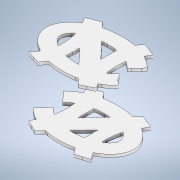
# Autodesk Inventor part: HousingLogoPositive
Saved by Autodesk Inventor 2020 (Build 240168000, 168)
## iProperties
Created: 2019-09-04
Part Number: HousingLogoPositive
Material: Generic
Document SubType Name: Modeling
Designer: Eric
Density: 1 g/cm^3
Appearance: White
Author: Eric
Autodesk Inventor part; units mm, degrees
note: some values were not read from the file. Chosen so that the rebuilt part matches the saved one: direction of "Hole1"; direction of "Hole2".
(part 1 of 2)
sketch "Sketch1" plane through (0, 0, 0) normal (0, 0, 1) x (1, 0, 0)
  arc A0 (31.8897, -7.6835) -> (33.4645, -6.1087) centre (31.8897, -6.1087) ccw projected
  line L0 (33.4645, 6.1087) -> (33.4645, -6.1087) projected
  arc A1 (33.4645, 6.1087) -> (31.8897, 7.6835) centre (31.8897, 6.1087) ccw projected
  line L1 (-31.8897, 7.6835) -> (31.8897, 7.6835) projected
  arc A2 (-31.8897, 7.6835) -> (-33.4645, 6.1087) centre (-31.8897, 6.1087) ccw projected
  line L2 (-33.4645, -6.1087) -> (-33.4645, 6.1087) projected
  arc A3 (-33.4645, -6.1087) -> (-31.8897, -7.6835) centre (-31.8897, -6.1087) ccw projected
  line L3 (31.8897, -7.6835) -> (-31.8897, -7.6835) projected
  circle A4 centre (-30.5562, 0) radius 1.524 projected
  circle A5 centre (30.5562, 0) radius 1.524 projected
  arc A6 (-24.5555, 6.9912) -> (-27.8573, 3.0561) centre (-24.5555, 3.6383) ccw projected
  line L4 (24.5555, 6.9912) -> (-24.5555, 6.9912) projected
  arc A7 (27.8573, 3.0561) -> (24.5555, 6.9912) centre (24.5555, 3.6383) ccw projected
  line L5 (26.5742, -4.2206) -> (27.8573, 3.0561) projected
  arc A8 (23.2724, -6.9912) -> (26.5742, -4.2206) centre (23.2724, -3.6383) ccw projected
  line L6 (-23.2724, -6.9912) -> (23.2724, -6.9912) projected
  arc A9 (-26.5742, -4.2206) -> (-23.2724, -6.9912) centre (-23.2724, -3.6383) ccw projected
  line L7 (-27.8573, 3.0561) -> (-26.5742, -4.2206) projected
  arc A10 (37.0645, 6.1087) -> (31.8897, 11.2835) centre (31.8897, 6.1087) ccw
  line L8 (37.0645, 6.1087) -> (37.0645, -6.1087)
  arc A11 (31.8897, -11.2835) -> (37.0645, -6.1087) centre (31.8897, -6.1087) ccw
  line L9 (31.8897, -11.2835) -> (-31.8897, -11.2835)
  arc A12 (-37.0645, -6.1087) -> (-31.8897, -11.2835) centre (-31.8897, -6.1087) ccw
  line L10 (-37.0645, -6.1087) -> (-37.0645, 6.1087)
  arc A13 (-31.8897, 11.2835) -> (-37.0645, 6.1087) centre (-31.8897, 6.1087) ccw
  line L11 (-31.8897, 11.2835) -> (31.8897, 11.2835)
  arc A14 (-24.5555, 7.3911) -> (-28.2512, 2.9867) centre (-24.5555, 3.6383) ccw
  line L12 (-24.5555, 7.3911) -> (24.5555, 7.3912)
  arc A15 (28.2512, 2.9867) -> (24.5555, 7.3912) centre (24.5555, 3.6383) ccw
  line L13 (28.2512, 2.9867) -> (26.9682, -4.29)
  arc A16 (23.2724, -7.3911) -> (26.9682, -4.29) centre (23.2724, -3.6383) ccw
  line L14 (23.2724, -7.3911) -> (-23.2724, -7.3912)
  arc A17 (-26.9682, -4.29) -> (-23.2724, -7.3912) centre (-23.2724, -3.6383) ccw
  line L15 (-26.9682, -4.29) -> (-28.2512, 2.9867)
  point P0 (0, 0)
  dimension "d0" = 3.6
  dimension "d1" = 0.4
  constraints: 16 end point, 16 point on circle, 8 centre point, 14 other
  measures "d0" distance between parallel lines of L1 L11
  measures "d1" distance between parallel lines of L4 L12
extrude "Extrusion1" add sketch "Sketch1" along normal blind 1.2 contours L3 A3 L2 A2 L1 A1 L0 A0 | L8 A11 L9 A12 L10 A13 L11 A10
sketch "Sketch2" plane through (0, 0, 0) normal (0, 0, -1) x (-1, 0, 0)
  arc A0 (-33.4645, -6.1087) -> (-31.8897, -7.6835) centre (-31.8897, -6.1087) ccw projected
  line L0 (-33.4645, 6.1087) -> (-33.4645, -6.1087) projected
  arc A1 (-31.8897, 7.6835) -> (-33.4645, 6.1087) centre (-31.8897, 6.1087) ccw projected
  line L1 (31.8897, 7.6835) -> (-31.8897, 7.6835) projected
  arc A2 (33.4645, 6.1087) -> (31.8897, 7.6835) centre (31.8897, 6.1087) ccw projected
  line L2 (33.4645, -6.1087) -> (33.4645, 6.1087) projected
  arc A3 (31.8897, -7.6835) -> (33.4645, -6.1087) centre (31.8897, -6.1087) ccw projected
  line L3 (-31.8897, -7.6835) -> (31.8897, -7.6835) projected
  circle A4 centre (30.5562, 0) radius 1.524 projected
  circle A5 centre (-30.5562, 0) radius 1.524 projected
  arc A6 (27.8573, 3.0561) -> (24.5555, 6.9912) centre (24.5555, 3.6383) ccw projected
  line L4 (-24.5555, 6.9912) -> (24.5555, 6.9912) projected
  arc A7 (-24.5555, 6.9912) -> (-27.8573, 3.0561) centre (-24.5555, 3.6383) ccw projected
  line L5 (-26.5742, -4.2206) -> (-27.8573, 3.0561) projected
  arc A8 (-26.5742, -4.2206) -> (-23.2724, -6.9912) centre (-23.2724, -3.6383) ccw projected
  line L6 (23.2724, -6.9912) -> (-23.2724, -6.9912) projected
  arc A9 (23.2724, -6.9912) -> (26.5742, -4.2206) centre (23.2724, -3.6383) ccw projected
  line L7 (27.8573, 3.0561) -> (26.5742, -4.2206) projected
  line L8 (37.0645, 6.1087) -> (37.0645, -6.1087) projected
  arc A10 (37.0645, 6.1087) -> (31.8897, 11.2835) centre (31.8897, 6.1087) ccw projected
  line L9 (-31.8897, 11.2835) -> (31.8897, 11.2835) projected
  arc A11 (-31.8897, 11.2835) -> (-37.0645, 6.1087) centre (-31.8897, 6.1087) ccw projected
  line L10 (-37.0645, -6.1087) -> (-37.0645, 6.1087) projected
  arc A12 (-37.0645, -6.1087) -> (-31.8897, -11.2835) centre (-31.8897, -6.1087) ccw projected
  line L11 (31.8897, -11.2835) -> (-31.8897, -11.2835) projected
  arc A13 (31.8897, -11.2835) -> (37.0645, -6.1087) centre (31.8897, -6.1087) ccw projected
  arc A14 (28.2512, 2.9867) -> (24.5555, 7.3911) centre (24.5555, 3.6383) ccw projected
  line L12 (26.9682, -4.29) -> (28.2512, 2.9867) projected
  arc A15 (23.2724, -7.3912) -> (26.9682, -4.29) centre (23.2724, -3.6383) ccw projected
  line L13 (-23.2724, -7.3911) -> (23.2724, -7.3912) projected
  arc A16 (-26.9682, -4.29) -> (-23.2724, -7.3911) centre (-23.2724, -3.6383) ccw projected
  line L14 (-28.2512, 2.9867) -> (-26.9682, -4.29) projected
  arc A17 (-24.5555, 7.3912) -> (-28.2512, 2.9867) centre (-24.5555, 3.6383) ccw projected
  line L15 (24.5555, 7.3911) -> (-24.5555, 7.3912) projected
  circle A18 centre (-30.5562, 0) radius 1.524 projected
  circle A19 centre (30.5562, 0) radius 1.524 projected
  arc A20 (-31.8897, 8.0835) -> (-33.8645, 6.1087) centre (-31.8897, 6.1087) ccw
  line L16 (-33.8645, 6.1087) -> (-33.8645, -6.1087)
  arc A21 (-33.8645, -6.1087) -> (-31.8897, -8.0835) centre (-31.8897, -6.1087) ccw
  line L17 (-31.8897, -8.0835) -> (31.8897, -8.0835)
  arc A22 (31.8897, -8.0835) -> (33.8645, -6.1087) centre (31.8897, -6.1087) ccw
  line L18 (33.8645, -6.1087) -> (33.8645, 6.1087)
  arc A23 (33.8645, 6.1087) -> (31.8897, 8.0835) centre (31.8897, 6.1087) ccw
  line L19 (31.8897, 8.0835) -> (-31.8897, 8.0835)
  point P0 (0, 0)
  dimension "d4" = 0.4
  constraints: 8 end point, 8 point on circle, 4 centre point, 7 other
  measures "d4" distance between parallel lines of L1 L19
extrude "Extrusion2" add sketch "Sketch2" along normal blind 1.6 contours L8 A13 L11 A12 L10 A11 L9 A10
sketch "Sketch3" plane through (0, 0, -1.6) normal (0, 0, -1) x (-1, 0, 0)
  line L0 (31.8897, 11.2835) -> (-31.8897, 11.2835) projected
  arc A0 (-31.8897, 11.2835) -> (-37.0645, 6.1087) centre (-31.8897, 6.1087) ccw projected
  line L1 (-37.0645, 6.1087) -> (-37.0645, -6.1087) projected
  arc A1 (-37.0645, -6.1087) -> (-31.8897, -11.2835) centre (-31.8897, -6.1087) ccw projected
  line L2 (-31.8897, -11.2835) -> (31.8897, -11.2835) projected
  arc A2 (31.8897, -11.2835) -> (37.0645, -6.1087) centre (31.8897, -6.1087) ccw projected
  line L3 (37.0645, -6.1087) -> (37.0645, 6.1087) projected
  arc A3 (37.0645, 6.1087) -> (31.8897, 11.2835) centre (31.8897, 6.1087) ccw projected
  arc A4 (-31.8897, 8.0835) -> (-33.8645, 6.1087) centre (-31.8897, 6.1087) ccw projected
  line L4 (-31.8897, 8.0835) -> (31.8897, 8.0835) projected
  arc A5 (33.8645, 6.1087) -> (31.8897, 8.0835) centre (31.8897, 6.1087) ccw projected
  line L5 (33.8645, 6.1087) -> (33.8645, -6.1087) projected
  arc A6 (31.8897, -8.0835) -> (33.8645, -6.1087) centre (31.8897, -6.1087) ccw projected
  line L6 (31.8897, -8.0835) -> (-31.8897, -8.0835) projected
  arc A7 (-33.8645, -6.1087) -> (-31.8897, -8.0835) centre (-31.8897, -6.1087) ccw projected
  line L7 (-33.8645, -6.1087) -> (-33.8645, 6.1087) projected
  circle A8 centre (-30.5562, 0) radius 1.524 projected
  line L8 (37.0645, 6.1087) -> (37.0645, -6.1087) projected
  arc A9 (31.8897, -11.2835) -> (37.0645, -6.1087) centre (31.8897, -6.1087) ccw projected
  line L9 (31.8897, -11.2835) -> (-31.8897, -11.2835) projected
  arc A10 (-37.0645, -6.1087) -> (-31.8897, -11.2835) centre (-31.8897, -6.1087) ccw projected
  line L10 (-37.0645, -6.1087) -> (-37.0645, 6.1087) projected
  arc A11 (-31.8897, 11.2835) -> (-37.0645, 6.1087) centre (-31.8897, 6.1087) ccw projected
  line L11 (-31.8897, 11.2835) -> (31.8897, 11.2835) projected
  arc A12 (37.0645, 6.1087) -> (31.8897, 11.2835) centre (31.8897, 6.1087) ccw projected
  arc A13 (28.2512, 2.9867) -> (24.5555, 7.3911) centre (24.5555, 3.6383) ccw projected
  line L12 (24.5555, 7.3911) -> (-24.5555, 7.3912) projected
  arc A14 (-24.5555, 7.3912) -> (-28.2512, 2.9867) centre (-24.5555, 3.6383) ccw projected
  line L13 (-28.2512, 2.9867) -> (-26.9682, -4.29) projected
  arc A15 (-26.9682, -4.29) -> (-23.2724, -7.3911) centre (-23.2724, -3.6383) ccw projected
  line L14 (-23.2724, -7.3911) -> (23.2724, -7.3912) projected
  arc A16 (23.2724, -7.3912) -> (26.9682, -4.29) centre (23.2724, -3.6383) ccw projected
  line L15 (26.9682, -4.29) -> (28.2512, 2.9867) projected
  circle A17 centre (-30.5562, 0) radius 1.524 projected
  circle A18 centre (30.5562, 0) radius 1.524 projected
  line L16 (-31.8897, -8.0835) -> (31.8897, -8.0835) projected
  arc A19 (28.2512, 2.9867) -> (24.5555, 7.3911) centre (24.5555, 3.6383) ccw projected
  line L17 (-23.2724, -7.3911) -> (23.2724, -7.3912) projected
  arc A20 (23.2724, -7.3912) -> (26.9682, -4.29) centre (23.2724, -3.6383) ccw projected
  point P0 (0, 0)
ref_plane "Work Plane1" through (20.4432, -5.693, -21.5638) normal (0, 0, 1) x (1, 0, 0)
extrude "Extrusion3" add sketch "Sketch3" along normal up to surface (19.9638 mm away) contours A3 L3 A2 L2 A1 L1 A0 L0 | L4 A5 L5 A6 L6 A7 L7 A4
sketch "Sketch4" plane through (31.8897, -11.2835, -21.5638) normal (0, 0, -1) x (-1, 0, 0)
  circle A0 centre (1.3335, 11.2835) radius 1.524 projected
  circle A1 centre (62.4459, 11.2835) radius 1.524 projected
  point P0 (31.8897, 11.2835)
  constraints: 2 coincident
hole "Hole1" at (-30.5562, 0, -21.5638) at (30.5562, 0, -21.5638) direction (0, 0, 1) diameter 3.2 depth 19.9638
ref_plane "Work Plane2" through (-21.3801, -2.5043, -26.2897) normal (0, -0.0871557, -0.9961947) x (1, 0, 0)
sketch "Sketch6" plane through (-21.3801, -2.5043, -26.2897) normal (0, -0.0871557, -0.9961947) x (1, 0, 0)
  arc A0 (-0.0392, 3.5884) -> (-0.8476, 1.4884) centre (1.375, 1.8384) ccw projected
  line L0 (-0.8476, 1.4884) -> (-0.325, 1.4884) projected
  line L1 (-0.325, 1.4884) -> (-0.325, 0.4134) projected
  line L2 (-0.325, 0.4134) -> (0, 0.0884) projected
  line L3 (0, 0.0884) -> (2.75, 0.0884) projected
  line L4 (2.75, 0.0884) -> (3.075, 0.4134) projected
  line L5 (3.075, 0.4134) -> (3.075, 1.4884) projected
  line L6 (3.075, 1.4884) -> (3.5976, 1.4884) projected
  arc A1 (3.5976, 1.4884) -> (2.7892, 3.5884) centre (1.375, 1.8384) ccw projected
  line L7 (-0.0392, 3.5884) -> (2.7892, 3.5884) projected
  circle A2 centre (1.375, 1.8384) radius 1.55 projected
  arc A3 (7.6685, -1.9054) -> (8.4769, 0.1946) centre (6.2543, -0.1554) ccw projected
  line L8 (8.4769, 0.1946) -> (7.9543, 0.1946) projected
  line L9 (7.9543, 0.1946) -> (7.9543, 1.2696) projected
  line L10 (7.9543, 1.2696) -> (7.6293, 1.5946) projected
  line L11 (7.6293, 1.5946) -> (4.8793, 1.5946) projected
  line L12 (4.8793, 1.5946) -> (4.5543, 1.2696) projected
  line L13 (4.5543, 1.2696) -> (4.5543, 0.1946) projected
  line L14 (4.5543, 0.1946) -> (4.0316, 0.1946) projected
  arc A4 (4.0316, 0.1946) -> (4.84, -1.9054) centre (6.2543, -0.1554) ccw projected
  line L15 (7.6685, -1.9054) -> (4.84, -1.9054) projected
  circle A5 centre (6.2543, -0.1554) radius 1.55 projected
  arc A6 (9.7193, 3.5884) -> (8.9109, 1.4884) centre (11.1335, 1.8384) ccw projected
  line L16 (8.9109, 1.4884) -> (9.4335, 1.4884) projected
  line L17 (9.4335, 1.4884) -> (9.4335, 0.4134) projected
  line L18 (9.4335, 0.4134) -> (9.7585, 0.0884) projected
  line L19 (9.7585, 0.0884) -> (12.5085, 0.0884) projected
  line L20 (12.5085, 0.0884) -> (12.8335, 0.4134) projected
  line L21 (12.8335, 0.4134) -> (12.8335, 1.4884) projected
  line L22 (12.8335, 1.4884) -> (13.3561, 1.4884) projected
  arc A7 (13.3561, 1.4884) -> (12.5477, 3.5884) centre (11.1335, 1.8384) ccw projected
  line L23 (9.7193, 3.5884) -> (12.5477, 3.5884) projected
  circle A8 centre (11.1335, 1.8384) radius 1.55 projected
  arc A9 (17.427, -1.9054) -> (18.2354, 0.1946) centre (16.0128, -0.1554) ccw projected
  line L24 (18.2354, 0.1946) -> (17.7128, 0.1946) projected
  line L25 (17.7128, 0.1946) -> (17.7128, 1.2696) projected
  line L26 (17.7128, 1.2696) -> (17.3878, 1.5946) projected
  line L27 (17.3878, 1.5946) -> (14.6378, 1.5946) projected
  line L28 (14.6378, 1.5946) -> (14.3128, 1.2696) projected
  line L29 (14.3128, 1.2696) -> (14.3128, 0.1946) projected
  line L30 (14.3128, 0.1946) -> (13.7902, 0.1946) projected
  arc A10 (13.7902, 0.1946) -> (14.5986, -1.9054) centre (16.0128, -0.1554) ccw projected
  line L31 (17.427, -1.9054) -> (14.5986, -1.9054) projected
  circle A11 centre (16.0128, -0.1554) radius 1.55 projected
  arc A12 (19.4778, 3.5884) -> (18.6694, 1.4884) centre (20.892, 1.8384) ccw projected
  line L32 (18.6694, 1.4884) -> (19.192, 1.4884) projected
  line L33 (19.192, 1.4884) -> (19.192, 0.4134) projected
  line L34 (19.192, 0.4134) -> (19.517, 0.0884) projected
  line L35 (19.517, 0.0884) -> (22.267, 0.0884) projected
  line L36 (22.267, 0.0884) -> (22.592, 0.4134) projected
  line L37 (22.592, 0.4134) -> (22.592, 1.4884) projected
  line L38 (22.592, 1.4884) -> (23.1147, 1.4884) projected
  arc A13 (23.1147, 1.4884) -> (22.3063, 3.5884) centre (20.892, 1.8384) ccw projected
  line L39 (19.4778, 3.5884) -> (22.3063, 3.5884) projected
  circle A14 centre (20.892, 1.8384) radius 1.55 projected
  arc A15 (27.1855, -1.9054) -> (27.9939, 0.1946) centre (25.7713, -0.1554) ccw projected
  line L40 (27.9939, 0.1946) -> (27.4713, 0.1946) projected
  line L41 (27.4713, 0.1946) -> (27.4713, 1.2696) projected
  line L42 (27.4713, 1.2696) -> (27.1463, 1.5946) projected
  line L43 (27.1463, 1.5946) -> (24.3963, 1.5946) projected
  line L44 (24.3963, 1.5946) -> (24.0713, 1.2696) projected
  line L45 (24.0713, 1.2696) -> (24.0713, 0.1946) projected
  line L46 (24.0713, 0.1946) -> (23.5487, 0.1946) projected
  arc A16 (23.5487, 0.1946) -> (24.3571, -1.9054) centre (25.7713, -0.1554) ccw projected
  line L47 (27.1855, -1.9054) -> (24.3571, -1.9054) projected
  circle A17 centre (25.7713, -0.1554) radius 1.55 projected
  arc A18 (29.2363, 3.5884) -> (28.4279, 1.4884) centre (30.6506, 1.8384) ccw projected
  line L48 (28.4279, 1.4884) -> (28.9506, 1.4884) projected
  line L49 (28.9506, 1.4884) -> (28.9506, 0.4134) projected
  line L50 (28.9506, 0.4134) -> (29.2756, 0.0884) projected
  line L51 (29.2756, 0.0884) -> (32.0256, 0.0884) projected
  line L52 (32.0256, 0.0884) -> (32.3506, 0.4134) projected
  line L53 (32.3506, 0.4134) -> (32.3506, 1.4884) projected
  line L54 (32.3506, 1.4884) -> (32.8732, 1.4884) projected
  arc A19 (32.8732, 1.4884) -> (32.0648, 3.5884) centre (30.6506, 1.8384) ccw projected
  line L55 (29.2363, 3.5884) -> (32.0648, 3.5884) projected
  circle A20 centre (30.6506, 1.8384) radius 1.55 projected
  arc A21 (36.944, -1.9054) -> (37.7524, 0.1946) centre (35.5298, -0.1554) ccw projected
  line L56 (37.7524, 0.1946) -> (37.2298, 0.1946) projected
  line L57 (37.2298, 0.1946) -> (37.2298, 1.2696) projected
  line L58 (37.2298, 1.2696) -> (36.9048, 1.5946) projected
  line L59 (36.9048, 1.5946) -> (34.1548, 1.5946) projected
  line L60 (34.1548, 1.5946) -> (33.8298, 1.2696) projected
  line L61 (33.8298, 1.2696) -> (33.8298, 0.1946) projected
  line L62 (33.8298, 0.1946) -> (33.3072, 0.1946) projected
  arc A22 (33.3072, 0.1946) -> (34.1156, -1.9054) centre (35.5298, -0.1554) ccw projected
  line L63 (36.944, -1.9054) -> (34.1156, -1.9054) projected
  circle A23 centre (35.5298, -0.1554) radius 1.55 projected
  arc A24 (38.9949, 3.5884) -> (38.1865, 1.4884) centre (40.4091, 1.8384) ccw projected
  line L64 (38.1865, 1.4884) -> (38.7091, 1.4884) projected
  line L65 (38.7091, 1.4884) -> (38.7091, 0.4134) projected
  line L66 (38.7091, 0.4134) -> (39.0341, 0.0884) projected
  line L67 (39.0341, 0.0884) -> (41.7841, 0.0884) projected
  line L68 (41.7841, 0.0884) -> (42.1091, 0.4134) projected
  line L69 (42.1091, 0.4134) -> (42.1091, 1.4884) projected
  line L70 (42.1091, 1.4884) -> (42.6317, 1.4884) projected
  arc A25 (42.6317, 1.4884) -> (41.8233, 3.5884) centre (40.4091, 1.8384) ccw projected
  line L71 (38.9949, 3.5884) -> (41.8233, 3.5884) projected
  circle A26 centre (40.4091, 1.8384) radius 1.55 projected
  arc A27 (46.7026, -1.9054) -> (47.511, 0.1946) centre (45.2883, -0.1554) ccw projected
  line L72 (47.511, 0.1946) -> (46.9883, 0.1946) projected
  line L73 (46.9883, 0.1946) -> (46.9883, 1.2696) projected
  line L74 (46.9883, 1.2696) -> (46.6633, 1.5946) projected
  line L75 (46.6633, 1.5946) -> (43.9133, 1.5946) projected
  line L76 (43.9133, 1.5946) -> (43.5883, 1.2696) projected
  line L77 (43.5883, 1.2696) -> (43.5883, 0.1946) projected
  line L78 (43.5883, 0.1946) -> (43.0657, 0.1946) projected
  arc A28 (43.0657, 0.1946) -> (43.8741, -1.9054) centre (45.2883, -0.1554) ccw projected
  line L79 (46.7026, -1.9054) -> (43.8741, -1.9054) projected
  circle A29 centre (45.2883, -0.1554) radius 1.55 projected
  line L80 (22.6421, 0.2446) -> (22.6421, 1.4384) projected
  line L81 (22.6421, 0.2446) -> (24.0213, 0.2446) projected
  line L82 (24.0213, 0.2446) -> (24.0213, 1.4384) projected
  line L83 (22.6421, 1.4384) -> (24.0213, 1.4384) projected
  line L84 (27.5213, 0.2446) -> (27.5213, 1.4384) projected
  line L85 (27.5213, 0.2446) -> (28.9006, 0.2446) projected
  line L86 (28.9006, 0.2446) -> (28.9006, 1.4384) projected
  line L87 (27.5213, 1.4384) -> (28.9006, 1.4384) projected
  line L88 (37.2799, 0.2446) -> (37.2799, 1.4384) projected
  line L89 (37.2799, 0.2446) -> (38.6591, 0.2446) projected
  line L90 (38.6591, 0.2446) -> (38.6591, 1.4384) projected
  line L91 (37.2799, 1.4384) -> (38.6591, 1.4384) projected
  line L92 (47.0384, 0.2446) -> (47.0384, 1.4384) projected
  line L93 (47.0384, 0.2446) -> (48.0885, 0.2446) projected
  line L94 (48.0885, 0.2446) -> (48.0885, 1.4384) projected
  line L95 (47.0384, 1.4384) -> (48.0885, 1.4384) projected
  line L96 (8.0043, 0.2446) -> (8.0043, 1.4384) projected
  line L97 (8.0043, 0.2446) -> (9.3835, 0.2446) projected
  line L98 (9.3835, 0.2446) -> (9.3835, 1.4384) projected
  line L99 (8.0043, 1.4384) -> (9.3835, 1.4384) projected
  line L100 (-1.425, 0.2446) -> (-1.425, 1.4384) projected
  line L101 (-1.425, 0.2446) -> (-0.375, 0.2446) projected
  line L102 (-0.375, 0.2446) -> (-0.375, 1.4384) projected
  line L103 (-1.425, 1.4384) -> (-0.375, 1.4384) projected
  line L104 (3.125, 0.2446) -> (3.125, 1.4384) projected
  line L105 (3.125, 0.2446) -> (4.5043, 0.2446) projected
  line L106 (4.5043, 0.2446) -> (4.5043, 1.4384) projected
  line L107 (3.125, 1.4384) -> (4.5043, 1.4384) projected
  line L108 (17.7628, 0.2446) -> (17.7628, 1.4384) projected
  line L109 (17.7628, 0.2446) -> (19.1421, 0.2446) projected
  line L110 (19.1421, 0.2446) -> (19.1421, 1.4384) projected
  line L111 (17.7628, 1.4384) -> (19.1421, 1.4384) projected
  line L112 (12.8835, 0.2446) -> (12.8835, 1.4384) projected
  line L113 (12.8835, 0.2446) -> (14.2628, 0.2446) projected
  line L114 (14.2628, 0.2446) -> (14.2628, 1.4384) projected
  line L115 (12.8835, 1.4384) -> (14.2628, 1.4384) projected
  line L116 (42.1591, 0.2446) -> (42.1591, 1.4384) projected
  line L117 (42.1591, 0.2446) -> (43.5384, 0.2446) projected
  line L118 (43.5384, 0.2446) -> (43.5384, 1.4384) projected
  line L119 (42.1591, 1.4384) -> (43.5384, 1.4384) projected
  line L120 (32.4006, 0.2446) -> (32.4006, 1.4384) projected
  line L121 (32.4006, 0.2446) -> (33.7799, 0.2446) projected
  line L122 (33.7799, 0.2446) -> (33.7799, 1.4384) projected
  line L123 (32.4006, 1.4384) -> (33.7799, 1.4384) projected
  arc A30 (-0.1742, 3.9884) -> (-1.1667, 1.0884) centre (1.375, 1.8384) ccw
  line L124 (-0.1742, 3.9884) -> (2.9242, 3.9884)
  arc A31 (3.9167, 1.0884) -> (2.9242, 3.9884) centre (1.375, 1.8384) ccw
  line L125 (3.9167, 1.0884) -> (3.475, 1.0884)
  line L126 (3.475, 1.0884) -> (3.475, 0.2478)
  line L127 (3.475, 0.2478) -> (2.9157, -0.3116)
  line L128 (2.9157, -0.3116) -> (-0.1657, -0.3116)
  line L129 (-0.1657, -0.3116) -> (-0.725, 0.2478)
  line L130 (-0.725, 0.2478) -> (-0.725, 1.0884)
  line L131 (-0.725, 1.0884) -> (-1.1667, 1.0884)
  arc A32 (3.7126, 0.5946) -> (4.7051, -2.3054) centre (6.2543, -0.1554) ccw
  line L132 (3.7126, 0.5946) -> (4.1543, 0.5946)
  line L133 (4.1543, 0.5946) -> (4.1543, 1.4353)
  line L134 (4.1543, 1.4353) -> (4.7136, 1.9946)
  line L135 (4.7136, 1.9946) -> (7.7949, 1.9946)
  line L136 (7.7949, 1.9946) -> (8.3543, 1.4353)
  line L137 (8.3543, 1.4353) -> (8.3543, 0.5946)
  line L138 (8.3543, 0.5946) -> (8.7959, 0.5946)
  arc A33 (7.8035, -2.3054) -> (8.7959, 0.5946) centre (6.2543, -0.1554) ccw
  line L139 (7.8035, -2.3054) -> (4.7051, -2.3054)
  arc A34 (9.5843, 3.9884) -> (8.5919, 1.0884) centre (11.1335, 1.8384) ccw
  line L140 (9.5843, 3.9884) -> (12.6827, 3.9884)
  arc A35 (13.6752, 1.0884) -> (12.6827, 3.9884) centre (11.1335, 1.8384) ccw
  line L141 (13.6752, 1.0884) -> (13.2335, 1.0884)
  line L142 (13.2335, 1.0884) -> (13.2335, 0.2478)
  line L143 (13.2335, 0.2478) -> (12.6742, -0.3116)
  line L144 (12.6742, -0.3116) -> (9.5928, -0.3116)
  line L145 (9.5928, -0.3116) -> (9.0335, 0.2478)
  line L146 (9.0335, 0.2478) -> (9.0335, 1.0884)
  line L147 (9.0335, 1.0884) -> (8.5919, 1.0884)
  arc A36 (13.4711, 0.5946) -> (14.4636, -2.3054) centre (16.0128, -0.1554) ccw
  line L148 (13.4711, 0.5946) -> (13.9128, 0.5946)
  line L149 (13.9128, 0.5946) -> (13.9128, 1.4353)
  line L150 (13.9128, 1.4353) -> (14.4721, 1.9946)
  line L151 (14.4721, 1.9946) -> (17.5535, 1.9946)
  line L152 (17.5535, 1.9946) -> (18.1128, 1.4353)
  line L153 (18.1128, 1.4353) -> (18.1128, 0.5946)
  line L154 (18.1128, 0.5946) -> (18.5544, 0.5946)
  arc A37 (17.562, -2.3054) -> (18.5544, 0.5946) centre (16.0128, -0.1554) ccw
  line L155 (17.562, -2.3054) -> (14.4636, -2.3054)
  arc A38 (23.4337, 1.0884) -> (22.4412, 3.9884) centre (20.892, 1.8384) ccw
  line L156 (23.4337, 1.0884) -> (22.992, 1.0884)
  line L157 (22.992, 1.0884) -> (22.992, 0.2478)
  line L158 (22.992, 0.2478) -> (22.4327, -0.3116)
  line L159 (22.4327, -0.3116) -> (19.3514, -0.3116)
  line L160 (19.3514, -0.3116) -> (18.792, 0.2478)
  line L161 (18.792, 0.2478) -> (18.792, 1.0884)
  line L162 (18.792, 1.0884) -> (18.3504, 1.0884)
  arc A39 (19.3428, 3.9884) -> (18.3504, 1.0884) centre (20.892, 1.8384) ccw
  line L163 (19.3428, 3.9884) -> (22.4412, 3.9884)
  arc A40 (23.2296, 0.5946) -> (24.2221, -2.3054) centre (25.7713, -0.1554) ccw
  line L164 (23.2296, 0.5946) -> (23.6713, 0.5946)
  line L165 (23.6713, 0.5946) -> (23.6713, 1.4353)
  line L166 (23.6713, 1.4353) -> (24.2306, 1.9946)
  line L167 (24.2306, 1.9946) -> (27.312, 1.9946)
  line L168 (27.312, 1.9946) -> (27.8713, 1.4353)
  line L169 (27.8713, 1.4353) -> (27.8713, 0.5946)
  line L170 (27.8713, 0.5946) -> (28.313, 0.5946)
  arc A41 (27.3205, -2.3054) -> (28.313, 0.5946) centre (25.7713, -0.1554) ccw
  line L171 (27.3205, -2.3054) -> (24.2221, -2.3054)
  arc A42 (29.1014, 3.9884) -> (28.1089, 1.0884) centre (30.6506, 1.8384) ccw
  line L172 (29.1014, 3.9884) -> (32.1998, 3.9884)
  arc A43 (33.1922, 1.0884) -> (32.1998, 3.9884) centre (30.6506, 1.8384) ccw
  line L173 (33.1922, 1.0884) -> (32.7506, 1.0884)
  line L174 (32.7506, 1.0884) -> (32.7506, 0.2478)
  line L175 (32.7506, 0.2478) -> (32.1912, -0.3116)
  line L176 (32.1912, -0.3116) -> (29.1099, -0.3116)
  line L177 (29.1099, -0.3116) -> (28.5506, 0.2478)
  line L178 (28.5506, 0.2478) -> (28.5506, 1.0884)
  line L179 (28.5506, 1.0884) -> (28.1089, 1.0884)
  arc A44 (32.9882, 0.5946) -> (33.9806, -2.3054) centre (35.5298, -0.1554) ccw
  line L180 (32.9882, 0.5946) -> (33.4298, 0.5946)
  line L181 (33.4298, 0.5946) -> (33.4298, 1.4353)
  line L182 (33.4298, 1.4353) -> (33.9891, 1.9946)
  line L183 (33.9891, 1.9946) -> (37.0705, 1.9946)
  line L184 (37.0705, 1.9946) -> (37.6298, 1.4353)
  line L185 (37.6298, 1.4353) -> (37.6298, 0.5946)
  line L186 (37.6298, 0.5946) -> (38.0715, 0.5946)
  arc A45 (37.079, -2.3054) -> (38.0715, 0.5946) centre (35.5298, -0.1554) ccw
  line L187 (37.079, -2.3054) -> (33.9806, -2.3054)
  arc A46 (38.8599, 3.9884) -> (37.8674, 1.0884) centre (40.4091, 1.8384) ccw
  line L188 (38.8599, 3.9884) -> (41.9583, 3.9884)
  arc A47 (42.9507, 1.0884) -> (41.9583, 3.9884) centre (40.4091, 1.8384) ccw
  line L189 (42.9507, 1.0884) -> (42.5091, 1.0884)
  line L190 (42.5091, 1.0884) -> (42.5091, 0.2478)
  line L191 (42.5091, 0.2478) -> (41.9498, -0.3116)
  line L192 (41.9498, -0.3116) -> (38.8684, -0.3116)
  line L193 (38.8684, -0.3116) -> (38.3091, 0.2478)
  line L194 (38.3091, 0.2478) -> (38.3091, 1.0884)
  line L195 (38.3091, 1.0884) -> (37.8674, 1.0884)
  arc A48 (42.7467, 0.5946) -> (43.7391, -2.3054) centre (45.2883, -0.1554) ccw
  line L196 (42.7467, 0.5946) -> (43.1883, 0.5946)
  line L197 (43.1883, 0.5946) -> (43.1883, 1.4353)
  line L198 (43.1883, 1.4353) -> (43.7477, 1.9946)
  line L199 (43.7477, 1.9946) -> (46.829, 1.9946)
  line L200 (46.829, 1.9946) -> (47.3883, 1.4353)
  line L201 (47.3883, 1.4353) -> (47.3883, 0.5946)
  line L202 (47.3883, 0.5946) -> (47.83, 0.5946)
  arc A49 (46.8375, -2.3054) -> (47.83, 0.5946) centre (45.2883, -0.1554) ccw
  line L203 (46.8375, -2.3054) -> (43.7391, -2.3054)
  line L204 (-1.425, 0.2446) -> (48.0885, 0.2446)
  line L205 (48.0885, 0.2446) -> (48.0885, 1.4384)
  line L206 (48.0885, 1.4384) -> (-1.425, 1.4384)
  line L207 (-1.425, 1.4384) -> (-1.425, 0.2446)
  line L208 (48.4885, -0.1554) -> (-1.825, -0.1554)
  line L209 (-1.825, -0.1554) -> (-1.825, 1.8384)
  line L210 (-1.825, 1.8384) -> (48.4885, 1.8384)
  line L211 (48.4885, 1.8384) -> (48.4885, -0.1554)
  point P0 (21.3801, -0.2035)
  point P1 (28.0006, 1.8384)
  point P2 (27.4682, 1.8384)
  point P3 (24.0744, 1.8384)
  point P4 (23.542, 1.8384)
  point P5 (18.242, 1.8384)
  point P6 (17.7097, 1.8384)
  point P7 (14.3159, 1.8384)
  point P8 (13.7835, 1.8384)
  point P9 (8.4835, 1.8384)
  point P10 (7.9511, 1.8384)
  point P11 (4.5574, 1.8384)
  point P12 (4.025, 1.8384)
  point P13 (-1.275, 1.8384)
  point P14 (-0.3219, -0.1554)
  point P15 (3.0719, -0.1554)
  point P16 (3.6043, -0.1554)
  point P17 (8.9043, -0.1554)
  point P18 (9.4366, -0.1554)
  point P19 (12.8304, -0.1554)
  point P20 (13.3628, -0.1554)
  point P21 (18.6628, -0.1554)
  point P22 (19.1952, -0.1554)
  point P23 (22.5889, -0.1554)
  point P24 (23.1213, -0.1554)
  point P25 (28.4213, -0.1554)
  point P26 (28.9537, -0.1554)
  point P27 (32.3474, -0.1554)
  point P28 (32.8798, -0.1554)
  point P29 (38.1798, -0.1554)
  point P30 (38.7122, -0.1554)
  point P31 (42.106, -0.1554)
  point P32 (42.6383, -0.1554)
  point P33 (47.9383, -0.1554)
  point P34 (46.9852, 1.8384)
  point P35 (43.5915, 1.8384)
  point P36 (43.0591, 1.8384)
  point P37 (37.7591, 1.8384)
  point P38 (37.2267, 1.8384)
  point P39 (33.8329, 1.8384)
  point P40 (33.3006, 1.8384)
  point P41 (27.8713, 1.8384)
  point P42 (23.6713, 1.8384)
  dimension "d18" = 0.4
  dimension "d19" = 0.4
  constraints: 172 end point, 40 point on circle, 20 centre point, 12 parallel, 1 horizontal, 1 perpendicular, 1 vertical, 99 other
  measures "d18" distance between parallel lines of L7 L124
  measures "d19" distance between parallel lines of L207 L209
sketch "Sketch7" plane through (31.8897, 11.2835, -21.5638) normal (0, 0, -1) x (-1, 0, 0)
  circle A0 centre (62.4459, -11.2835) radius 1.6 projected
  circle A1 centre (1.3335, -11.2835) radius 1.6 projected
  arc A2 (7.3343, -3.8923) -> (3.6385, -8.2968) centre (7.3342, -7.6452) ccw projected
  line L0 (7.3343, -3.8923) -> (56.4451, -3.8924) projected
  arc A3 (60.1409, -8.2968) -> (56.4451, -3.8924) centre (56.4451, -7.6452) ccw projected
  line L1 (60.1409, -8.2968) -> (58.8579, -15.5735) projected
  arc A4 (55.1621, -18.6747) -> (58.8579, -15.5735) centre (55.1621, -14.9219) ccw projected
  line L2 (55.1621, -18.6747) -> (8.6173, -18.6746) projected
  arc A5 (4.9215, -15.5735) -> (8.6173, -18.6746) centre (8.6173, -14.9219) ccw projected
  line L3 (4.9215, -15.5735) -> (3.6385, -8.2968) projected
  arc A6 (63.7794, -22.567) -> (68.9542, -17.3922) centre (63.7794, -17.3922) ccw projected
  line L4 (68.9542, -17.3922) -> (68.9542, -5.1748) projected
  arc A7 (68.9542, -5.1748) -> (63.7794, 0) centre (63.7794, -5.1748) ccw projected
  line L5 (63.7794, 0) -> (0, 0) projected
  arc A8 (0, 0) -> (-5.1748, -5.1748) centre (0, -5.1748) ccw projected
  line L6 (-5.1748, -5.1748) -> (-5.1748, -17.3922) projected
  arc A9 (-5.1748, -17.3922) -> (0, -22.567) centre (0, -17.3922) ccw projected
  line L7 (0, -22.567) -> (63.7794, -22.567) projected
  circle A10 centre (1.3335, -11.2835) radius 1.524
  circle A11 centre (62.4459, -11.2835) radius 1.524
  point P0 (31.8897, -11.2835)
  constraints: 2 centre point, 4 other
ref_plane "Work Plane3" through (22.2277, 2.6133, -26.3842) normal (0, 0.0871557, -0.9961947) x (-1, 0, 0)
sketch "Sketch8" plane through (22.2277, 2.6133, -26.3842) normal (0, 0.0871557, -0.9961947) x (-1, 0, 0)
  arc A0 (25.2047, 3.479) -> (24.3963, 1.379) centre (26.6189, 1.729) ccw projected
  line L0 (24.3963, 1.379) -> (24.9189, 1.379) projected
  line L1 (24.9189, 1.379) -> (24.9189, 0.304) projected
  line L2 (24.9189, 0.304) -> (25.2439, -0.021) projected
  line L3 (25.2439, -0.021) -> (27.9939, -0.021) projected
  line L4 (27.9939, -0.021) -> (28.3189, 0.304) projected
  line L5 (28.3189, 0.304) -> (28.3189, 1.379) projected
  line L6 (28.3189, 1.379) -> (28.8415, 1.379) projected
  arc A1 (28.8415, 1.379) -> (28.0331, 3.479) centre (26.6189, 1.729) ccw projected
  line L7 (25.2047, 3.479) -> (28.0331, 3.479) projected
  circle A2 centre (26.6189, 1.729) radius 1.55 projected
  arc A3 (23.1539, -2.0148) -> (23.9623, 0.0852) centre (21.7397, -0.2648) ccw projected
  line L8 (23.9623, 0.0852) -> (23.4397, 0.0852) projected
  line L9 (23.4397, 0.0852) -> (23.4397, 1.1602) projected
  line L10 (23.4397, 1.1602) -> (23.1147, 1.4852) projected
  line L11 (23.1147, 1.4852) -> (20.3647, 1.4852) projected
  line L12 (20.3647, 1.4852) -> (20.0397, 1.1602) projected
  line L13 (20.0397, 1.1602) -> (20.0397, 0.0852) projected
  line L14 (20.0397, 0.0852) -> (19.517, 0.0852) projected
  arc A4 (19.517, 0.0852) -> (20.3254, -2.0148) centre (21.7397, -0.2648) ccw projected
  line L15 (23.1539, -2.0148) -> (20.3254, -2.0148) projected
  circle A5 centre (21.7397, -0.2648) radius 1.55 projected
  arc A6 (15.4462, 3.479) -> (14.6378, 1.379) centre (16.8604, 1.729) ccw projected
  line L16 (14.6378, 1.379) -> (15.1604, 1.379) projected
  line L17 (15.1604, 1.379) -> (15.1604, 0.304) projected
  line L18 (15.1604, 0.304) -> (15.4854, -0.021) projected
  line L19 (15.4854, -0.021) -> (18.2354, -0.021) projected
  line L20 (18.2354, -0.021) -> (18.5604, 0.304) projected
  line L21 (18.5604, 0.304) -> (18.5604, 1.379) projected
  line L22 (18.5604, 1.379) -> (19.083, 1.379) projected
  arc A7 (19.083, 1.379) -> (18.2746, 3.479) centre (16.8604, 1.729) ccw projected
  line L23 (15.4462, 3.479) -> (18.2746, 3.479) projected
  circle A8 centre (16.8604, 1.729) radius 1.55 projected
  arc A9 (13.3953, -2.0148) -> (14.2037, 0.0852) centre (11.9811, -0.2648) ccw projected
  line L24 (14.2037, 0.0852) -> (13.6811, 0.0852) projected
  line L25 (13.6811, 0.0852) -> (13.6811, 1.1602) projected
  line L26 (13.6811, 1.1602) -> (13.3561, 1.4852) projected
  line L27 (13.3561, 1.4852) -> (10.6061, 1.4852) projected
  line L28 (10.6061, 1.4852) -> (10.2811, 1.1602) projected
  line L29 (10.2811, 1.1602) -> (10.2811, 0.0852) projected
  line L30 (10.2811, 0.0852) -> (9.7585, 0.0852) projected
  arc A10 (9.7585, 0.0852) -> (10.5669, -2.0148) centre (11.9811, -0.2648) ccw projected
  line L31 (13.3953, -2.0148) -> (10.5669, -2.0148) projected
  circle A11 centre (11.9811, -0.2648) radius 1.55 projected
  arc A12 (5.6877, 3.479) -> (4.8793, 1.379) centre (7.1019, 1.729) ccw projected
  line L32 (4.8793, 1.379) -> (5.4019, 1.379) projected
  line L33 (5.4019, 1.379) -> (5.4019, 0.304) projected
  line L34 (5.4019, 0.304) -> (5.7269, -0.021) projected
  line L35 (5.7269, -0.021) -> (8.4769, -0.021) projected
  line L36 (8.4769, -0.021) -> (8.8019, 0.304) projected
  line L37 (8.8019, 0.304) -> (8.8019, 1.379) projected
  line L38 (8.8019, 1.379) -> (9.3245, 1.379) projected
  arc A13 (9.3245, 1.379) -> (8.5161, 3.479) centre (7.1019, 1.729) ccw projected
  line L39 (5.6877, 3.479) -> (8.5161, 3.479) projected
  circle A14 centre (7.1019, 1.729) radius 1.55 projected
  arc A15 (3.6368, -2.0148) -> (4.4452, 0.0852) centre (2.2226, -0.2648) ccw projected
  line L40 (4.4452, 0.0852) -> (3.9226, 0.0852) projected
  line L41 (3.9226, 0.0852) -> (3.9226, 1.1602) projected
  line L42 (3.9226, 1.1602) -> (3.5976, 1.4852) projected
  line L43 (3.5976, 1.4852) -> (0.8476, 1.4852) projected
  line L44 (0.8476, 1.4852) -> (0.5226, 1.1602) projected
  line L45 (0.5226, 1.1602) -> (0.5226, 0.0852) projected
  line L46 (0.5226, 0.0852) -> (0, 0.0852) projected
  arc A16 (0, 0.0852) -> (0.8084, -2.0148) centre (2.2226, -0.2648) ccw projected
  line L47 (3.6368, -2.0148) -> (0.8084, -2.0148) projected
  circle A17 centre (2.2226, -0.2648) radius 1.55 projected
  arc A18 (44.7217, 3.479) -> (43.9133, 1.379) centre (46.136, 1.729) ccw projected
  line L48 (43.9133, 1.379) -> (44.436, 1.379) projected
  line L49 (44.436, 1.379) -> (44.436, 0.304) projected
  line L50 (44.436, 0.304) -> (44.761, -0.021) projected
  line L51 (44.761, -0.021) -> (47.511, -0.021) projected
  line L52 (47.511, -0.021) -> (47.836, 0.304) projected
  line L53 (47.836, 0.304) -> (47.836, 1.379) projected
  line L54 (47.836, 1.379) -> (48.3586, 1.379) projected
  arc A19 (48.3586, 1.379) -> (47.5502, 3.479) centre (46.136, 1.729) ccw projected
  line L55 (44.7217, 3.479) -> (47.5502, 3.479) projected
  circle A20 centre (46.136, 1.729) radius 1.55 projected
  arc A21 (42.6709, -2.0148) -> (43.4793, 0.0852) centre (41.2567, -0.2648) ccw projected
  line L56 (43.4793, 0.0852) -> (42.9567, 0.0852) projected
  line L57 (42.9567, 0.0852) -> (42.9567, 1.1602) projected
  line L58 (42.9567, 1.1602) -> (42.6317, 1.4852) projected
  line L59 (42.6317, 1.4852) -> (39.8817, 1.4852) projected
  line L60 (39.8817, 1.4852) -> (39.5567, 1.1602) projected
  line L61 (39.5567, 1.1602) -> (39.5567, 0.0852) projected
  line L62 (39.5567, 0.0852) -> (39.0341, 0.0852) projected
  arc A22 (39.0341, 0.0852) -> (39.8425, -2.0148) centre (41.2567, -0.2648) ccw projected
  line L63 (42.6709, -2.0148) -> (39.8425, -2.0148) projected
  circle A23 centre (41.2567, -0.2648) radius 1.55 projected
  arc A24 (34.9632, 3.479) -> (34.1548, 1.379) centre (36.3774, 1.729) ccw projected
  line L64 (34.1548, 1.379) -> (34.6774, 1.379) projected
  line L65 (34.6774, 1.379) -> (34.6774, 0.304) projected
  line L66 (34.6774, 0.304) -> (35.0024, -0.021) projected
  line L67 (35.0024, -0.021) -> (37.7524, -0.021) projected
  line L68 (37.7524, -0.021) -> (38.0774, 0.304) projected
  line L69 (38.0774, 0.304) -> (38.0774, 1.379) projected
  line L70 (38.0774, 1.379) -> (38.6, 1.379) projected
  arc A25 (38.6, 1.379) -> (37.7916, 3.479) centre (36.3774, 1.729) ccw projected
  line L71 (34.9632, 3.479) -> (37.7916, 3.479) projected
  circle A26 centre (36.3774, 1.729) radius 1.55 projected
  arc A27 (32.9124, -2.0148) -> (33.7208, 0.0852) centre (31.4982, -0.2648) ccw projected
  line L72 (33.7208, 0.0852) -> (33.1982, 0.0852) projected
  line L73 (33.1982, 0.0852) -> (33.1982, 1.1602) projected
  line L74 (33.1982, 1.1602) -> (32.8732, 1.4852) projected
  line L75 (32.8732, 1.4852) -> (30.1232, 1.4852) projected
  line L76 (30.1232, 1.4852) -> (29.7982, 1.1602) projected
  line L77 (29.7982, 1.1602) -> (29.7982, 0.0852) projected
  line L78 (29.7982, 0.0852) -> (29.2756, 0.0852) projected
  arc A28 (29.2756, 0.0852) -> (30.084, -2.0148) centre (31.4982, -0.2648) ccw projected
  line L79 (32.9124, -2.0148) -> (30.084, -2.0148) projected
  circle A29 centre (31.4982, -0.2648) radius 1.55 projected
  line L80 (47.886, 0.1352) -> (47.886, 1.329) projected
  line L81 (47.886, 0.1352) -> (48.9361, 0.1352) projected
  line L82 (48.9361, 0.1352) -> (48.9361, 1.329) projected
  line L83 (47.886, 1.329) -> (48.9361, 1.329) projected
  line L84 (-0.5774, 0.1352) -> (-0.5774, 1.329) projected
  line L85 (-0.5774, 0.1352) -> (0.4726, 0.1352) projected
  line L86 (0.4726, 0.1352) -> (0.4726, 1.329) projected
  line L87 (-0.5774, 1.329) -> (0.4726, 1.329) projected
  line L88 (3.9726, 0.1352) -> (3.9726, 1.329) projected
  line L89 (3.9726, 0.1352) -> (5.3519, 0.1352) projected
  line L90 (5.3519, 0.1352) -> (5.3519, 1.329) projected
  line L91 (3.9726, 1.329) -> (5.3519, 1.329) projected
  line L92 (8.8519, 0.1352) -> (8.8519, 1.329) projected
  line L93 (8.8519, 0.1352) -> (10.2312, 0.1352) projected
  line L94 (10.2312, 0.1352) -> (10.2312, 1.329) projected
  line L95 (8.8519, 1.329) -> (10.2312, 1.329) projected
  line L96 (13.7312, 0.1352) -> (13.7312, 1.329) projected
  line L97 (13.7312, 0.1352) -> (15.1104, 0.1352) projected
  line L98 (15.1104, 0.1352) -> (15.1104, 1.329) projected
  line L99 (13.7312, 1.329) -> (15.1104, 1.329) projected
  line L100 (23.4897, 0.1352) -> (23.4897, 1.329) projected
  line L101 (23.4897, 0.1352) -> (24.8689, 0.1352) projected
  line L102 (24.8689, 0.1352) -> (24.8689, 1.329) projected
  line L103 (23.4897, 1.329) -> (24.8689, 1.329) projected
  line L104 (28.3689, 0.1352) -> (28.3689, 1.329) projected
  line L105 (28.3689, 0.1352) -> (29.7482, 0.1352) projected
  line L106 (29.7482, 0.1352) -> (29.7482, 1.329) projected
  line L107 (28.3689, 1.329) -> (29.7482, 1.329) projected
  line L108 (33.2482, 0.1352) -> (33.2482, 1.329) projected
  line L109 (33.2482, 0.1352) -> (34.6275, 0.1352) projected
  line L110 (34.6275, 0.1352) -> (34.6275, 1.329) projected
  line L111 (33.2482, 1.329) -> (34.6275, 1.329) projected
  line L112 (43.0067, 0.1352) -> (43.0067, 1.329) projected
  line L113 (43.0067, 0.1352) -> (44.386, 0.1352) projected
  line L114 (44.386, 0.1352) -> (44.386, 1.329) projected
  line L115 (43.0067, 1.329) -> (44.386, 1.329) projected
  line L116 (38.1275, 0.1352) -> (38.1275, 1.329) projected
  line L117 (38.1275, 0.1352) -> (39.5067, 0.1352) projected
  line L118 (39.5067, 0.1352) -> (39.5067, 1.329) projected
  line L119 (38.1275, 1.329) -> (39.5067, 1.329) projected
  line L120 (48.9361, 1.329) -> (-0.5774, 1.329)
  line L121 (-0.5774, 1.329) -> (-0.5774, 0.1352)
  line L122 (-0.5774, 0.1352) -> (48.9361, 0.1352)
  line L123 (48.9361, 0.1352) -> (48.9361, 1.329)
  arc A30 (-0.319, 0.4852) -> (0.6734, -2.4148) centre (2.2226, -0.2648) ccw
  line L124 (-0.319, 0.4852) -> (0.1226, 0.4852)
  line L125 (0.1226, 0.4852) -> (0.1226, 1.3259)
  line L126 (0.1226, 1.3259) -> (0.6819, 1.8852)
  line L127 (0.6819, 1.8852) -> (3.7633, 1.8852)
  line L128 (3.7633, 1.8852) -> (4.3226, 1.3259)
  line L129 (4.3226, 1.3259) -> (4.3226, 0.4852)
  line L130 (4.3226, 0.4852) -> (4.7643, 0.4852)
  arc A31 (3.7718, -2.4148) -> (4.7643, 0.4852) centre (2.2226, -0.2648) ccw
  line L131 (3.7718, -2.4148) -> (0.6734, -2.4148)
  line L132 (49.3361, -0.2648) -> (-0.9774, -0.2648)
  line L133 (-0.9774, -0.2648) -> (-0.9774, 1.729)
  line L134 (-0.9774, 1.729) -> (49.3361, 1.729)
  line L135 (49.3361, 1.729) -> (49.3361, -0.2648)
  arc A32 (5.5527, 3.879) -> (4.5602, 0.979) centre (7.1019, 1.729) ccw
  line L136 (5.5527, 3.879) -> (8.6511, 3.879)
  arc A33 (9.6435, 0.979) -> (8.6511, 3.879) centre (7.1019, 1.729) ccw
  line L137 (9.6435, 0.979) -> (9.2019, 0.979)
  line L138 (9.2019, 0.979) -> (9.2019, 0.1383)
  line L139 (9.2019, 0.1383) -> (8.6426, -0.421)
  line L140 (8.6426, -0.421) -> (5.5612, -0.421)
  line L141 (5.5612, -0.421) -> (5.0019, 0.1383)
  line L142 (5.0019, 0.1383) -> (5.0019, 0.979)
  line L143 (5.0019, 0.979) -> (4.5602, 0.979)
  arc A34 (13.5303, -2.4148) -> (14.5228, 0.4852) centre (11.9811, -0.2648) ccw
  line L144 (13.5303, -2.4148) -> (10.4319, -2.4148)
  arc A35 (9.4395, 0.4852) -> (10.4319, -2.4148) centre (11.9811, -0.2648) ccw
  line L145 (9.4395, 0.4852) -> (9.8811, 0.4852)
  line L146 (9.8811, 0.4852) -> (9.8811, 1.3259)
  line L147 (9.8811, 1.3259) -> (10.4404, 1.8852)
  line L148 (10.4404, 1.8852) -> (13.5218, 1.8852)
  line L149 (13.5218, 1.8852) -> (14.0811, 1.3259)
  line L150 (14.0811, 1.3259) -> (14.0811, 0.4852)
  line L151 (14.0811, 0.4852) -> (14.5228, 0.4852)
  arc A36 (15.3112, 3.879) -> (14.3187, 0.979) centre (16.8604, 1.729) ccw
  line L152 (15.3112, 3.879) -> (18.4096, 3.879)
  arc A37 (19.402, 0.979) -> (18.4096, 3.879) centre (16.8604, 1.729) ccw
  line L153 (19.402, 0.979) -> (18.9604, 0.979)
  line L154 (18.9604, 0.979) -> (18.9604, 0.1383)
  line L155 (18.9604, 0.1383) -> (18.4011, -0.421)
  line L156 (18.4011, -0.421) -> (15.3197, -0.421)
  line L157 (15.3197, -0.421) -> (14.7604, 0.1383)
  line L158 (14.7604, 0.1383) -> (14.7604, 0.979)
  line L159 (14.7604, 0.979) -> (14.3187, 0.979)
  arc A38 (23.2888, -2.4148) -> (24.2813, 0.4852) centre (21.7397, -0.2648) ccw
  line L160 (23.2888, -2.4148) -> (20.1905, -2.4148)
  arc A39 (19.198, 0.4852) -> (20.1905, -2.4148) centre (21.7397, -0.2648) ccw
  line L161 (19.198, 0.4852) -> (19.6397, 0.4852)
  line L162 (19.6397, 0.4852) -> (19.6397, 1.3259)
  line L163 (19.6397, 1.3259) -> (20.199, 1.8852)
  line L164 (20.199, 1.8852) -> (23.2803, 1.8852)
  line L165 (23.2803, 1.8852) -> (23.8397, 1.3259)
  line L166 (23.8397, 1.3259) -> (23.8397, 0.4852)
  line L167 (23.8397, 0.4852) -> (24.2813, 0.4852)
  arc A40 (25.0697, 3.879) -> (24.0773, 0.979) centre (26.6189, 1.729) ccw
  line L168 (25.0697, 3.879) -> (28.1681, 3.879)
  arc A41 (29.1606, 0.979) -> (28.1681, 3.879) centre (26.6189, 1.729) ccw
  line L169 (29.1606, 0.979) -> (28.7189, 0.979)
  line L170 (28.7189, 0.979) -> (28.7189, 0.1383)
  line L171 (28.7189, 0.1383) -> (28.1596, -0.421)
  line L172 (28.1596, -0.421) -> (25.0782, -0.421)
  line L173 (25.0782, -0.421) -> (24.5189, 0.1383)
  line L174 (24.5189, 0.1383) -> (24.5189, 0.979)
  line L175 (24.5189, 0.979) -> (24.0773, 0.979)
  arc A42 (33.0474, -2.4148) -> (34.0398, 0.4852) centre (31.4982, -0.2648) ccw
  line L176 (33.0474, -2.4148) -> (29.949, -2.4148)
  arc A43 (28.9565, 0.4852) -> (29.949, -2.4148) centre (31.4982, -0.2648) ccw
  line L177 (28.9565, 0.4852) -> (29.3982, 0.4852)
  line L178 (29.3982, 0.4852) -> (29.3982, 1.3259)
  line L179 (29.3982, 1.3259) -> (29.9575, 1.8852)
  line L180 (29.9575, 1.8852) -> (33.0389, 1.8852)
  line L181 (33.0389, 1.8852) -> (33.5982, 1.3259)
  line L182 (33.5982, 1.3259) -> (33.5982, 0.4852)
  line L183 (33.5982, 0.4852) -> (34.0398, 0.4852)
  arc A44 (34.8282, 3.879) -> (33.8358, 0.979) centre (36.3774, 1.729) ccw
  line L184 (34.8282, 3.879) -> (37.9266, 3.879)
  arc A45 (38.9191, 0.979) -> (37.9266, 3.879) centre (36.3774, 1.729) ccw
  line L185 (38.9191, 0.979) -> (38.4774, 0.979)
  line L186 (38.4774, 0.979) -> (38.4774, 0.1383)
  line L187 (38.4774, 0.1383) -> (37.9181, -0.421)
  line L188 (37.9181, -0.421) -> (34.8367, -0.421)
  line L189 (34.8367, -0.421) -> (34.2774, 0.1383)
  line L190 (34.2774, 0.1383) -> (34.2774, 0.979)
  line L191 (34.2774, 0.979) -> (33.8358, 0.979)
  arc A46 (42.8059, -2.4148) -> (43.7983, 0.4852) centre (41.2567, -0.2648) ccw
  line L192 (42.8059, -2.4148) -> (39.7075, -2.4148)
  arc A47 (38.715, 0.4852) -> (39.7075, -2.4148) centre (41.2567, -0.2648) ccw
  line L193 (38.715, 0.4852) -> (39.1567, 0.4852)
  line L194 (39.1567, 0.4852) -> (39.1567, 1.3259)
  line L195 (39.1567, 1.3259) -> (39.716, 1.8852)
  line L196 (39.716, 1.8852) -> (42.7974, 1.8852)
  line L197 (42.7974, 1.8852) -> (43.3567, 1.3259)
  line L198 (43.3567, 1.3259) -> (43.3567, 0.4852)
  line L199 (43.3567, 0.4852) -> (43.7983, 0.4852)
  arc A48 (44.5868, 3.879) -> (43.5943, 0.979) centre (46.136, 1.729) ccw
  line L200 (44.5868, 3.879) -> (47.6851, 3.879)
  arc A49 (48.6776, 0.979) -> (47.6851, 3.879) centre (46.136, 1.729) ccw
  line L201 (48.6776, 0.979) -> (48.236, 0.979)
  line L202 (48.236, 0.979) -> (48.236, 0.1383)
  line L203 (48.236, 0.1383) -> (47.6766, -0.421)
  line L204 (47.6766, -0.421) -> (44.5953, -0.421)
  line L205 (44.5953, -0.421) -> (44.036, 0.1383)
  line L206 (44.036, 0.1383) -> (44.036, 0.979)
  line L207 (44.036, 0.979) -> (43.5943, 0.979)
  point P0 (22.2277, -0.3039)
  point P1 (44.4391, -0.2648)
  point P2 (47.8328, -0.2648)
  point P3 (48.786, 1.729)
  point P4 (43.486, 1.729)
  point P5 (39.0274, 1.729)
  point P6 (33.7274, 1.729)
  point P7 (33.1951, 1.729)
  point P8 (29.8013, 1.729)
  point P9 (29.2689, 1.729)
  point P10 (23.9689, 1.729)
  point P11 (23.4365, 1.729)
  point P12 (20.0428, 1.729)
  point P13 (19.5104, 1.729)
  point P14 (14.2104, 1.729)
  point P15 (13.678, 1.729)
  point P16 (10.2842, 1.729)
  point P17 (9.7519, 1.729)
  point P18 (4.4519, 1.729)
  point P19 (3.9195, 1.729)
  point P20 (0.5257, 1.729)
  point P21 (-0.4274, -0.2648)
  point P22 (4.8726, -0.2648)
  point P23 (5.405, -0.2648)
  point P24 (8.7988, -0.2648)
  point P25 (9.3311, -0.2648)
  point P26 (14.6311, -0.2648)
  point P27 (15.1635, -0.2648)
  point P28 (18.5573, -0.2648)
  point P29 (19.0897, -0.2648)
  point P30 (24.3897, -0.2648)
  point P31 (24.922, -0.2648)
  point P32 (28.3158, -0.2648)
  point P33 (28.8482, -0.2648)
  point P34 (34.1482, -0.2648)
  point P35 (34.6805, -0.2648)
  point P36 (38.0743, -0.2648)
  point P37 (38.6067, -0.2648)
  point P38 (43.9067, -0.2648)
  point P39 (39.5598, 1.729)
  point P40 (42.9536, 1.729)
  point P41 (23.8397, 1.729)
  point P42 (19.6397, 1.729)
  point P43 (14.0811, 1.729)
  point P44 (9.8811, 1.729)
  point P45 (0.1257, 1.329)
  point P46 (-0.397, 0.1352)
  dimension "d24" = 0.4
  dimension "d25" = 0.4
  constraints: 172 end point, 40 point on circle, 20 centre point, 12 parallel, 1 horizontal, 1 perpendicular, 1 vertical, 99 other
  measures "d24" distance between parallel lines of L55 L200
  measures "d25" distance between parallel lines of L135 L82
extrude "Extrusion4" add sketch "Sketch7" along normal up to surface (4.4131 mm away) contours A0 | A1 | L0 A3 L1 A4 L2 A5 L3 A2 | L7 A9 L6 A8 L5 A7 L4 A6
extrude "Extrusion5" cut sketch "Sketch6" against normal through all both and the other way through all
extrude "Extrusion6" cut sketch "Sketch8" against normal through all
sketch "Sketch12" plane through (-31.8897, 11.2835, 1.2) normal (0, 1, 0) x (1, 0, 0)
  line L0 (64.0459, 2.8) -> (64.0459, 22.7638) projected
  line L1 (-0.2665, 2.8) -> (-0.2665, 22.7638) projected
  line L2 (2.8575, 27.177) -> (-0.1905, 27.177) projected
  line L3 (-0.1905, 22.7638) -> (2.8575, 22.7638) projected
  line L4 (63.9699, 27.177) -> (60.9219, 27.177) projected
  line L5 (60.9219, 22.7638) -> (63.9699, 22.7638) projected
  line L6 (64.0459, 12.7819) -> (-0.2665, 12.7819)
  line L7 (64.0459, 2.8) -> (68.9542, 2.8)
  line L8 (68.9542, 27.177) -> (68.9542, 0) projected
  line L9 (66.5001, 2.8) -> (66.5001, 0)
  line L10 (-0.2665, 22.7638) -> (-5.1748, 22.7638)
  line L11 (-5.1748, 0) -> (-5.1748, 27.177) projected
  line L12 (-2.7207, 22.7638) -> (-2.7207, 27.1421)
  point P0 (31.8897, 1.2)
  point P1 (66.5001, 12.7819)
  point P2 (-2.7207, 12.7819)
  constraints: 10 end point, 6 point on line, 4 midpoint, 2 horizontal, 2 vertical
hole "Hole2" at (-34.6104, 11.2835, -11.5819) direction (0, -1, 0) diameter 2.2098 depth 11.2835 clearance for "Socket Head Cap Screw" size "M2" standard "Ansi Metric M Profile"
hole "Hole3" at (-34.6104, 11.2835, -11.5819) direction (0, -1, 0) diameter 1.567 end through all thread size "M2x0.4" class "6H" standard "ANSI Metric M Profile"
hole "Hole4" at (-34.6104, 11.2835, -11.5819) direction (0, -1, 0) diameter 4 depth 7
mirror "Mirror2" about plane through (0, 0, 0) normal (1, 0, 0) of "Hole2", "Hole3", "Hole4"
sketch "Sketch16" plane through (31.8897, 11.2835, -25.977) normal (0, 0, -1) x (-1, 0, 0)
  line L0 (4.7812, -13.6045) -> (58.9982, -13.6045)
  line L1 (58.9982, -13.6045) -> (58.9982, -8.9716)
  line L2 (58.9982, -8.9716) -> (4.7812, -8.9716)
  line L3 (4.7812, -8.9716) -> (4.7812, -13.6045)
  line L4 (55.0947, -13.6045) -> (55.0947, -15.6059) projected
  line L5 (58.9982, -8.9716) -> (8.6847, -8.9716) projected
  line L6 (4.7812, -13.6045) -> (55.0947, -13.6045) projected
  line L7 (4.7812, -15.6059) -> (4.7812, -13.6045) projected
  line L8 (58.9982, -6.9702) -> (58.9982, -8.9716) projected
  point P0 (15.067, -8.9716)
  point P1 (14.5346, -8.9716)
  point P2 (14.5576, -13.6045)
  point P3 (15.0899, -13.6045)
  constraints: 8 end point, 4 collinear, 2 parallel, 1 horizontal, 1 perpendicular
surface extrude "ExtrusionSrf3" sketch "Sketch16" against normal through all shown no curves L1 L2 L3 L0
sketch "Sketch21" plane through (0, 0, 1.2) normal (0, 0, 1) x (1, 0, 0)
  circle A0 centre (-30.5562, 0) radius 1.524 projected
  circle A1 centre (30.5562, 0) radius 1.524 projected
  point P0 (0, 0)
hole "Hole9" at (-30.5562, 0, 1.2) at (30.5562, 0, 1.2) direction (0, 0, 1) diameter 4.4 depth 22.7638
sketch "Sketch24" plane through (31.8897, 11.2835, -25.977) normal (0, 0, -1) x (-1, 0, 0)
  point P0 (31.8897, -11.2835)
  point P1 (31.8897, -11.2835)
  constraints: 1 coincident